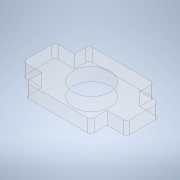
# Autodesk Inventor part: Laser-Slot-Term-Beam
Saved by Autodesk Inventor 2021 (Build 250183000, 183)
## iProperties
Created: 2020-06-23
Part Number: Laser-Slot-Term-Beam
Material: Acrylic, Clear
Document SubType Name: Modeling
Designer: lucas
Density: 1.19 g/cm^3
Appearance: Transparent - Clear
Project: 4Wire-Laser
Author: lucas
Revision Number: RLS_001
Autodesk Inventor part; units mm, degrees
ref_plane "YZ Plane" through (0, 0, 0) normal (1, 0, 0) x (0, 1, 0)
ref_plane "XZ Plane" through (0, 0, 0) normal (0, 1, 0) x (-1, 0, 0)
ref_plane "XY Plane" through (0, 0, 0) normal (0, 0, 1) x (1, 0, 0)
sketch "Sketch1" plane through (0, 0, 0) normal (0, 1, 0) x (-1, 0, 0)
  line L0 (1, -19.5) -> (19, -19.5)
  circle A0 centre (10, -10.25) radius 5.65
  line L1 (1, 0) -> (19, 0)
  line L2 (20, -1) -> (20, -5) construction
  line L3 (20, -5) -> (25, -5)
  line L4 (26, -6) -> (26, -14)
  line L5 (25, -15) -> (20, -15)
  line L6 (20, -18.5) -> (20, -15)
  line L7 (20, -5) -> (20, -1)
  line L8 (0, -1) -> (0, -5)
  line L9 (0, -5) -> (-5, -5)
  line L10 (-6, -6) -> (-6, -14)
  line L11 (-5, -15) -> (0, -15)
  line L12 (0, -15) -> (0, -18.5)
  arc A1 (0, -18.5) -> (1, -19.5) centre (1, -18.5) ccw
  arc A2 (1, 0) -> (0, -1) centre (1, -1) ccw
  arc A3 (20, -1) -> (19, 0) centre (19, -1) ccw
  arc A4 (26, -6) -> (25, -5) centre (25, -6) ccw
  arc A5 (25, -15) -> (26, -14) centre (25, -14) ccw
  arc A6 (19, -19.5) -> (20, -18.5) centre (19, -18.5) ccw
  arc A7 (-5, -5) -> (-6, -6) centre (-5, -6) ccw
  arc A8 (-6, -14) -> (-5, -15) centre (-5, -14) ccw
  line L13 (10, -10.25) -> (26, -10.25) construction
  point P0 (0, 0)
  point P1 (-6, -15)
  point P2 (-6, -5)
  point P3 (20, -1)
  dimension "d5" = 1
  dimension "d6" = 1
  dimension "d9" = 1
  dimension "d10" = 11.3
  constraints: 28 end point, 16 point on circle, 16 tangent, 9 centre point, 7 point on line, 5 equal radius, 5 perpendicular, 2 horizontal, 2 parallel, 1 vertical
  measures "d5" radius of A1
  measures "d6" radius of A6
  measures "d9" radius of A7
  measures "d10" diameter of A0
extrude "Extrusion1" add sketch "Sketch1" along normal blind 4
body "Solid1"
